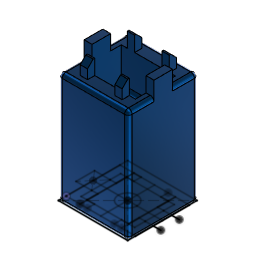
switchopen (Autodesk Fusion 360 design; units mm, degrees)
Autodesk Fusion 360 part; units mm, degrees
note: some values were not read from the file. Set by a fixed rule: which sketch regions a step uses.
sketch "Sketch1" plane through (0, 0, 0) normal (0, 0, 1) x (1, 0, 0)
  line L0 (0, 0) -> (18.62, 0)
  line L1 (18.62, 0) -> (18.62, 14.49)
  line L2 (18.62, 14.49) -> (0, 14.49)
  line L3 (0, 14.49) -> (0, 0)
  line L4 (9.31, 0) -> (9.31, 14.49)
  line L5 (0, 7.245) -> (18.62, 7.245)
  line L6 (2.1, 9.73) -> (-2.1, 9.73)
  line L7 (-2.1, 9.73) -> (-2.1, 4.76)
  line L8 (-2.1, 4.76) -> (2.1, 4.76)
  line L9 (2.1, 4.76) -> (2.1, 9.73)
  line L10 (2.1, 9.73) -> (-2.1, 4.76) construction
  line L11 (-2.1, 9.73) -> (2.1, 4.76) construction
  line L12 (3.72, 0) -> (3.72, 14.49)
  line L13 (3.72, 14.49) -> (5.66, 14.49)
  line L14 (5.66, 14.49) -> (5.66, 12.57)
  line L15 (5.66, 12.57) -> (3.72, 12.57)
  line L16 (3.72, 12.57) -> (3.72, 14.49)
  line L17 (5.66, 1.92) -> (3.72, 1.92)
  line L18 (3.72, 1.92) -> (3.72, 0)
  line L19 (5.66, 0) -> (5.66, 1.92)
  line L20 (16.52, 9.73) -> (20.72, 9.73)
  line L21 (16.52, 4.76) -> (16.52, 9.73)
  line L22 (20.72, 4.76) -> (16.52, 4.76)
  line L23 (12.96, 14.49) -> (12.96, 12.57)
  line L24 (12.96, 12.57) -> (14.9, 12.57)
  line L25 (14.9, 12.57) -> (14.9, 14.49)
  line L26 (12.96, 1.92) -> (14.9, 1.92)
  line L27 (12.96, 0) -> (12.96, 1.92)
  line L28 (14.9, 0) -> (14.9, 14.49)
  line L29 (3.72, 12.57) -> (14.9, 12.57)
  line L30 (14.9, 12.57) -> (14.9, 1.92)
  line L31 (14.9, 1.92) -> (3.72, 1.92)
  line L32 (3.72, 1.92) -> (3.72, 12.57)
  line L33 (2.1, 9.73) -> (3.72, 9.73)
  line L34 (3.72, 9.73) -> (3.72, 12.57)
  line L35 (3.72, 12.57) -> (2.1, 12.57)
  line L36 (2.1, 12.57) -> (2.1, 9.73)
  line L37 (2.1, 4.76) -> (3.72, 4.76)
  line L38 (3.72, 4.76) -> (3.72, 1.92)
  line L39 (3.72, 1.92) -> (2.1, 1.92)
  line L40 (2.1, 1.92) -> (2.1, 4.76)
  line L41 (14.9, 1.92) -> (16.52, 1.92)
  line L42 (16.52, 1.92) -> (16.52, 4.76)
  line L43 (16.52, 4.76) -> (14.9, 4.76)
  line L44 (14.9, 4.76) -> (14.9, 1.92)
  line L45 (16.52, 9.73) -> (14.9, 9.73)
  line L46 (14.9, 9.73) -> (14.9, 12.57)
  line L47 (14.9, 12.57) -> (16.52, 12.57)
  line L48 (16.52, 12.57) -> (16.52, 9.73)
  circle A0 centre (9.31, 7.245) radius 2.5
  line L49 (18.62, -2.065) -> (0, -2.065)
  line L50 (0, -2.065) -> (0, 16.555)
  line L51 (0, 16.555) -> (18.62, 16.555)
  line L52 (18.62, 16.555) -> (18.62, -2.065)
  line L53 (18.62, -2.065) -> (0, 16.555) construction
  line L54 (0, -2.065) -> (18.62, 16.555) construction
  point P0 (0, 7.245)
  point P1 (9.31, 7.245)
  dimension "d1" = 18.62
  dimension "d2" = 14.49
  dimension "d3" = 4.2
  dimension "d4" = 4.97
  dimension "d5" = -5.59
  dimension "d6" = 1.94
  dimension "d7" = 1.92
  dimension "d16" = 5
  dimension "d19" = 18.62
  dimension "d20" = 18.62
  constraint horizontal L0
  constraint vertical L1
  constraint horizontal L2
  constraint vertical L3
  constraint coincident L0.start L3.end
  constraint midpoint L0 L4.start
  constraint midpoint L2 L4.end
  constraint midpoint L3 P0
  constraint midpoint L1 L5.end
  constraint horizontal L6
  constraint perpendicular L6 L7
  constraint parallel L6 L8
  constraint parallel L7 L9
  constraint coincident L10 P0
  constraint coincident L11 P0
  constraint coincident P0 L5.start
  constraint horizontal L13
  constraint vertical L14
  constraint horizontal L15
  constraint vertical L16
  constraint symmetric L5 L12.end L12.start
  constraint symmetric L5 L13.end L19.start
  constraint symmetric L5 L14.end L17.start
  constraint symmetric L5 L15.end L17.end
  constraint symmetric L4 L6.start L20.start
  constraint symmetric L4 L6.end L20.end
  constraint symmetric L4 L7.end L22.start
  constraint symmetric L4 L8.end L21.start
  constraint symmetric L4 L12.start L28.start
  constraint symmetric L4 L12.end L25.end
  constraint symmetric L4 L13.end L23.start
  constraint symmetric L4 L14.end L23.end
  constraint symmetric L4 L15.end L24.end
  constraint symmetric L4 L17.start L26.start
  constraint symmetric L4 L17.end L26.end
  constraint symmetric L4 L19.start L27.start
  constraint horizontal L29
  constraint vertical L30
  constraint horizontal L31
  constraint vertical L32
  constraint horizontal L33
  constraint vertical L34
  constraint horizontal L35
  constraint vertical L36
  constraint horizontal L37
  constraint vertical L38
  constraint horizontal L39
  constraint vertical L40
  constraint horizontal L41
  constraint vertical L42
  constraint horizontal L43
  constraint vertical L44
  constraint horizontal L45
  constraint vertical L46
  constraint horizontal L47
  constraint vertical L48
  constraint midpoint L4 P1
  constraint horizontal L49
  constraint perpendicular L49 L50
  constraint parallel L49 L51
  constraint parallel L50 L52
  constraint coincident L53 P1
  constraint coincident L54 P1
  constraint coincident P1 A0.centre
  measures "d1" distance of L0.start L0.end
  measures "d2" distance of L0.start L2.end
  measures "d3" distance of L7.end L8.end
  measures "d4" distance of L6.end L7.end
  measures "d6" distance of L12.end L13.end
  measures "d7" distance of L12.end L15.end
  measures "d16" diameter of A0
  measures "d19" distance of L50.end L51.end
  measures "d20" distance of L49.end L50.end
extrude "Extrude1" add sketch "Sketch1" along normal blind 34 contours L0 L12 L17 L18 L19 L31 | L3 L5 L8 L9 L50 | L3 L5 L6 L9 L50 | L0 L26 L27 L28 L31 | L1 L5 L21 L22 L52 | L2 L12 L13 L14 L15 L16 L29 | L1 L5 L20 L21 L52 | L2 L23 L24 L25 L28 L29 makes body 1 at (13.6067, 0, 22.6667) makes body 2 at (5.0133, 14.49, 22.6667) makes body 3 at (18.62, 6.4167, 11.3333) makes body 4 at (4.3667, 0, 22.6667) makes body 5 at (0, 8.0733, 11.3333) makes body 6 at (14.2533, 14.49, 22.6667)
extrude "Extrude4" add sketch "Sketch1" along normal blind 30 contours L0 L3 L8 L12 L18 L39 L40 L50 | L0 L4 L19 L31 | L0 L4 L27 L31 | L2 L3 L6 L12 L16 L35 L36 L50 | L0 L1 L22 L28 L41 L42 L52 | L2 L4 L14 L29 | L1 L2 L20 L25 L28 L47 L48 L52 | L2 L4 L23 L29 bodies 1 2 3 4 5 6
extrude "Extrude5" add sketch "Sketch1" along normal blind 20 contours L12 L32 L37 L38 L39 L40 | L4 L5 L12 L17 L31 L32 L38 A0 | L5 L9 L12 L32 L37 | L5 L9 L12 L32 L33 | L4 L5 L26 L28 L30 L31 L44 A0 | L4 L5 L12 L15 L29 L32 L34 A0 | L12 L32 L33 L34 L35 L36 | L4 L5 A0 | L4 L5 A0 | L4 L5 A0 | L28 L30 L41 L42 L43 L44 | L5 L21 L28 L30 L43 | L4 L5 A0 | L4 L5 L24 L28 L29 L30 L46 A0 | L5 L21 L28 L30 L45 | L28 L30 L45 L46 L47 L48 bodies 1
extrude "Extrude6" add sketch "Sketch1" along normal blind 30 contours L0 L49 L50 L52 | L2 L13 L50 L51 L52 bodies 1
fillet "Fillet1" radius 1 4 edges at (18.62, 16.555, 15) (0, 16.555, 15) (0, -2.065, 15) (18.62, -2.065, 15) on bodies 1
fillet "Fillet2" radius 1 10 edges at (18.62, 12.6425, 30) (18.3271, 16.2621, 30) (9.31, 16.555, 30) (0.2929, 16.2621, 30) (0, 12.6425, 30) (0, 1.8475, 30) (0.2929, -1.7721, 30) (9.31, -2.065, 30) (18.3271, -1.7721, 30) (18.62, 1.8475, 30) on bodies 1
chamfer "Chamfer1" distance 1.5 angle 45 1 edges at (4.69, 0, 34) on bodies 1
chamfer "Chamfer2" distance 1.5 angle 45 1 edges at (13.93, 0, 34) on bodies 1
chamfer "Chamfer3" distance 1.5 angle 45 2 edges at (4.69, 14.49, 34) (13.93, 14.49, 34) on bodies 1
fillet "Fillet3" radius 1 4 edges at (9.31, 1.92, 20) (16.52, 7.245, 20) (2.1, 7.245, 20) (9.31, 12.57, 20) on bodies 1
fillet "Fillet4" radius 1 8 edges at (0.2929, -1.7721, 0) (0, 7.245, 0) (0.2929, 16.2621, 0) (9.31, 16.555, 0) (18.3271, 16.2621, 0) (18.62, 7.245, 0) (18.3271, -1.7721, 0) (9.31, -2.065, 0) on bodies 1
scale "Scale1" factor 1.01 about (0, -1.065, 29) bodies 1
